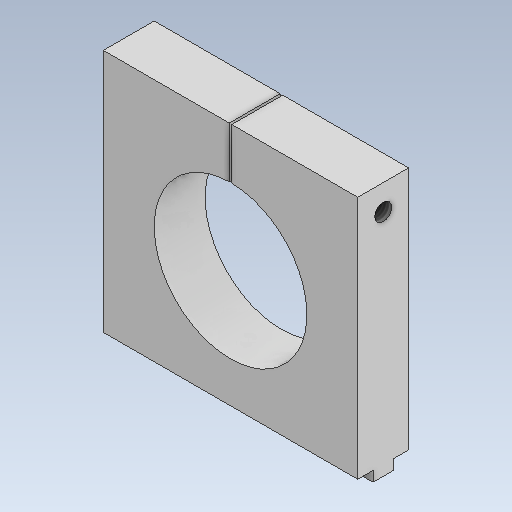
# Autodesk Inventor part: upperClamp
Saved by Autodesk Inventor 2021 (Build 250183000, 183)
## iProperties
Created: 2022-09-08
Part Number: upperClamp
Material: Generic
Document SubType Name: Modeling
Designer: szucs
Density: 1 g/cm^3
Appearance: Default
Author: szucs
Autodesk Inventor part; units mm, degrees
ref_plane "YZ Plane" through (0, 0, 0) normal (1, 0, 0) x (0, 1, 0)
ref_plane "XZ Plane" through (0, 0, 0) normal (0, 1, 0) x (-1, 0, 0)
ref_plane "XY Plane" through (0, 0, 0) normal (0, 0, 1) x (1, 0, 0)
sketch "Sketch1" plane through (0, 0, 0) normal (0, 0, 1) x (1, 0, 0)
  line L0 (0, 70) -> (0, -70) projected
  line L1 (-70, 0) -> (70, 0) projected
  line L2 (-50, 50) -> (50, 50)
  line L3 (50, 50) -> (50, -50)
  line L4 (50, -50) -> (-50, -50)
  line L5 (-50, -50) -> (-50, 50)
  circle A0 centre (0, 0) radius 30
  dimension "d0" = 100
  dimension "d1" = 100
  dimension "d2" = 60
  constraints: 8 end point, 2 parallel, 1 centre point, 1 coincident, 1 horizontal, 1 perpendicular, 2 other
  measures "d0" distance of L3.end L4.end
  measures "d1" distance of L2.end L3.end
  measures "d2" diameter of A0
extrude "Extrusion1" add sketch "Sketch1" along normal blind 20 contours L2 L3 L1 A0 L0 | L0 A0 L1 L5 L2 | L1 L3 L4 L0 A0 | A0 L0 L4 L5 L1
sketch "Sketch2" plane through (-50, -50, 0) normal (0, -1, 0) x (1, 0, 0)
  line L0 (20, 20) -> (20, 0) projected
  line L1 (0, 0) -> (100, 0) projected
  line L2 (100, 0) -> (100, 20) projected
  line L3 (0, 20) -> (100, 20) projected
  line L4 (0, 0) -> (0, 20) projected
  line L5 (80, 20) -> (80, 0) projected
  line L6 (0, 0) -> (0, 20) projected
  line L7 (0, 10) -> (100, 10)
  line L8 (0, 14) -> (100, 14)
  line L9 (0, 6) -> (100, 6)
  point P0 (50, 0)
  dimension "d5" = 4
  dimension "d6" = 4
  constraints: 6 end point, 2 midpoint, 2 parallel, 2 point on line
  measures "d5" distance between parallel lines of L7 L8
  measures "d6" distance between parallel lines of L7 L9
extrude "Extrusion2" cut sketch "Sketch2" against normal blind 4 contours L3 L5 L8 L0 | L0 L8 L4 L3 | L3 L2 L8 L5 | L9 L5 L1 L0 | L0 L1 L4 L9 | L9 L2 L1 L5
sketch "Sketch3" plane through (0, 0, 0) normal (0, 0, -1) x (-1, 0, 0)
  line L0 (0, -70) -> (0, 70) projected
  line L1 (0.5, -70) -> (0.5, 70)
  line L2 (-0.5, -70) -> (-0.5, 70)
  line L3 (-50, -46) -> (50, -46) projected
  line L4 (50, 50) -> (50, -46) projected
  line L5 (-50, 50) -> (50, 50) projected
  line L6 (-50, -46) -> (-50, 50) projected
  circle A0 centre (0, 0) radius 30 projected
  point P0 (0.5, 29.9958)
  point P1 (0.5, 50)
  point P2 (-0.5, 50)
  point P3 (-0.5, 29.9958)
  dimension "d9" = 0.5
  dimension "d10" = 0.5
  constraints: 4 end point, 2 parallel
  measures "d9" distance between parallel lines of L0 L1
  measures "d10" distance between parallel lines of L0 L2
extrude "Extrusion3" cut sketch "Sketch3" against normal through all contours A0 L2 L5 L0 | L0 L5 L1 A0
sketch "Sketch4" plane through (50, 50, 20) normal (1, 0, 0) x (0, 0, -1)
  line L0 (20, 0) -> (0, 0) projected
  line L1 (20, -96) -> (20, 0) projected
  point P0 (20, -50)
  point P1 (10, -10)
  dimension "d13" = 10
  dimension "d14" = 10
  measures "d13" distance from line of L0 point (10, -10)
  measures "d14" distance from line of L1 point (10, -10)
hole "Hole1" at (50, 40, 10) direction (-1, 0, 0) diameter 6.647 depth 110 tip angle 118 thread size "M8x1.25" class "6H" standard "ISO Metric profile"
sketch "Sketch5" plane through (-50, -50, 14) normal (0, -1, 0) x (1, 0, 0)
  line L0 (100, -14) -> (0, -14) projected
  line L1 (100, -8) -> (100, 0) projected
  point P0 (50, -14)
  point P1 (90, -4)
  dimension "d22" = 10
  dimension "d23" = 10
  measures "d22" distance from line of L0 point (90, -4)
  measures "d23" distance from line of L1 point (90, -4)
hole "Hole2" at (40, -50, 10) direction (0, 1, 0) diameter 6.647 depth 30 tip angle 118 thread size "M8x1.25" class "6H" standard "ISO Metric profile"
sketch "Sketch6" plane through (-50, -50, 14) normal (0, -1, 0) x (1, 0, 0)
  line L0 (0, -8) -> (0, 0) projected
  line L1 (100, -14) -> (0, -14) projected
  point P0 (50, -14)
  point P1 (10, -4)
  dimension "d31" = 10
  dimension "d32" = 10
  measures "d31" distance from line of L0 point (10, -4)
  measures "d32" distance from line of L1 point (10, -4)
hole "Hole3" at (-40, -50, 10) direction (0, 1, 0) diameter 6.647 depth 30 tip angle 118 thread size "M8x1.25" class "6H" standard "ISO Metric profile"
body "Solid1"
